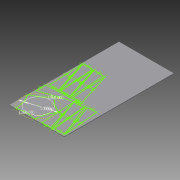
# Autodesk Inventor part: Birdhouse Board
Saved by Autodesk Inventor 2015 (Build 190159000, 159)
## iProperties
Created: 2018-03-09
Part Number: Birdhouse Board
Material: Generic
Document SubType Name: Modeling
Designer: Administrator
Density: 1 g/cm^3
Appearance: Default
Author: Administrator
Autodesk Inventor part; units mm, degrees
ref_plane "YZ Plane" through (0, 0, 0) normal (1, 0, 0) x (0, 1, 0)
ref_plane "XZ Plane" through (0, 0, 0) normal (0, 1, 0) x (-1, 0, 0)
ref_plane "XY Plane" through (0, 0, 0) normal (0, 0, 1) x (1, 0, 0)
sketch "Sketch1" plane through (0, 0, 0) normal (0, 1, 0) x (-1, 0, 0)
  line L0 (101.6, 169.3333) -> (-203.2, 169.3333)
  line L1 (-203.2, 169.3333) -> (-203.2, -440.2667)
  line L2 (-203.2, -440.2667) -> (101.6, -440.2667)
  line L3 (101.6, -440.2667) -> (101.6, 169.3333)
  point P0 (0, 0)
  dimension "d0" = 304.8
  dimension "d1" = 609.6
  constraints: 8 end point, 2 parallel, 1 horizontal, 1 perpendicular
  measures "d0" distance of L0.start L0.end
  measures "d1" distance of L0.end L1.end
extrude "Extrusion1" add sketch "Sketch1" along normal blind 3.175
sketch "Sketch2" plane through (0, 3.175, 0) normal (0, 1, 0) x (1, 0, 0)
  circle A0 centre (-15.875, -95.25) radius 63.5 construction
  circle A1 centre (-15.875, -95.25) radius 88.9 construction
  line L0 (-15.875, -6.35) -> (-53.1994, -43.8774)
  line L1 (-53.1994, -43.8774) -> (-100.4239, -67.7784)
  line L2 (-100.4239, -67.7784) -> (-76.2671, -114.8726)
  line L3 (-76.2671, -114.8726) -> (-68.1291, -167.1716)
  line L4 (-68.1291, -167.1716) -> (-15.875, -158.75)
  line L5 (36.3791, -167.1716) -> (-15.875, -158.75)
  line L6 (44.5171, -114.8726) -> (36.3791, -167.1716)
  line L7 (44.5171, -114.8726) -> (68.6739, -67.7784)
  line L8 (68.6739, -67.7784) -> (21.4494, -43.8774)
  line L9 (21.4494, -43.8774) -> (-15.875, -6.35)
  line L10 (122.7836, -165.1) -> (103.3018, -165.1)
  line L11 (103.3018, -168.275) -> (103.3018, -165.1)
  line L12 (95.6818, -168.275) -> (103.3018, -168.275)
  line L13 (95.6818, -165.1) -> (95.6818, -168.275)
  line L14 (73.025, -165.1) -> (95.6818, -165.1)
  line L15 (73.025, -165.1) -> (68.1796, -72.334)
  line L16 (68.1796, -72.334) -> (73.025, -165.1)
  line L17 (68.1796, -72.334) -> (71.3503, -72.1684)
  line L18 (71.3503, -72.1684) -> (70.9528, -64.5588)
  line L19 (70.9528, -64.5588) -> (71.3503, -72.1684)
  line L20 (70.9528, -64.5588) -> (67.7821, -64.7244)
  line L21 (67.7821, -64.7244) -> (70.9528, -64.5588)
  line L22 (67.7821, -64.7244) -> (63.2239, 22.5422)
  line L23 (67.7821, -64.7244) -> (63.2239, 22.5422)
  line L24 (63.2239, 22.5422) -> (90.9783, -64.8977)
  line L25 (90.9783, -64.8977) -> (63.2239, 22.5422)
  line L26 (90.9783, -64.8977) -> (87.9521, -65.8583)
  line L27 (87.9521, -65.8583) -> (90.2574, -73.1212)
  line L28 (90.2574, -73.1212) -> (93.2836, -72.1607)
  line L29 (90.2574, -73.1212) -> (93.2836, -72.1607)
  line L30 (93.2836, -72.1607) -> (122.7836, -165.1)
  line L31 (63.2239, 22.5422) -> (85.8673, 23.3211)
  line L32 (85.8673, 23.3211) -> (85.7582, 26.4942)
  line L33 (85.7582, 26.4942) -> (93.3737, 26.7562)
  line L34 (93.3737, 26.7562) -> (93.4828, 23.583)
  line L35 (93.4828, 23.583) -> (116.1262, 24.3619)
  line L36 (93.4828, 23.583) -> (116.1262, 24.3619)
  line L37 (116.1262, 24.3619) -> (124.1586, -68.1926)
  line L38 (124.1586, -68.1926) -> (116.1262, 24.3619)
  line L39 (124.1586, -68.1926) -> (127.3217, -67.9181)
  line L40 (127.3217, -67.9181) -> (127.9805, -75.5095)
  line L41 (127.3217, -67.9181) -> (127.9805, -75.5095)
  line L42 (127.9805, -75.5095) -> (124.8174, -75.784)
  line L43 (124.8174, -75.784) -> (132.8498, -168.3385)
  line L44 (124.8174, -75.784) -> (132.8498, -168.3385)
  line L45 (132.8498, -168.3385) -> (99.3425, -76.4774)
  line L46 (96.3597, -77.5654) -> (93.7485, -70.4068)
  line L47 (99.3425, -76.4774) -> (96.3597, -77.5654)
  line L48 (96.3597, -77.5654) -> (93.7485, -70.4068)
  line L49 (93.7485, -70.4068) -> (96.7313, -69.3188)
  line L50 (96.7313, -69.3188) -> (63.2239, 22.5422)
  line L51 (190.9567, -155.6753) -> (168.3382, -156.9913)
  line L52 (168.3382, -156.9913) -> (168.5226, -160.161)
  line L53 (168.5226, -160.161) -> (160.9155, -160.6036)
  line L54 (168.5226, -160.161) -> (160.9155, -160.6036)
  line L55 (160.9155, -160.6036) -> (160.731, -157.4339)
  line L56 (160.731, -157.4339) -> (138.1125, -158.75)
  line L57 (160.731, -157.4339) -> (138.1125, -158.75)
  line L58 (138.1125, -158.75) -> (127.8857, -66.4122)
  line L59 (127.8857, -66.4122) -> (138.1125, -158.75)
  line L60 (127.8857, -66.4122) -> (124.73, -66.7618)
  line L61 (124.73, -66.7618) -> (123.8912, -59.1881)
  line L62 (124.73, -66.7618) -> (123.8912, -59.1881)
  line L63 (123.8912, -59.1881) -> (127.0469, -58.8386)
  line L64 (127.0469, -58.8386) -> (116.8201, 33.4992)
  line L65 (127.0469, -58.8386) -> (116.8201, 33.4992)
  line L66 (116.8201, 33.4992) -> (152.4982, -57.5407)
  line L67 (155.4543, -56.3822) -> (158.2347, -63.4769)
  line L68 (152.4982, -57.5407) -> (155.4543, -56.3822)
  line L69 (155.4543, -56.3822) -> (158.2347, -63.4769)
  line L70 (158.2347, -63.4769) -> (155.2786, -64.6354)
  line L71 (155.2786, -64.6354) -> (190.9567, -155.6753)
  line L72 (155.2786, -64.6354) -> (190.9567, -155.6753)
  line L73 (190.9567, -155.6753) -> (168.3382, -156.9913)
  line L74 (168.3382, -156.9913) -> (168.5226, -160.161)
  line L75 (168.5226, -160.161) -> (160.9155, -160.6036)
  line L76 (168.5226, -160.161) -> (160.9155, -160.6036)
  line L77 (160.9155, -160.6036) -> (160.731, -157.4339)
  line L78 (160.731, -157.4339) -> (138.1125, -158.75)
  line L79 (160.731, -157.4339) -> (138.1125, -158.75)
  line L80 (138.1125, -158.75) -> (127.8857, -66.4122)
  line L81 (127.8857, -66.4122) -> (138.1125, -158.75)
  line L82 (127.8857, -66.4122) -> (124.73, -66.7618)
  line L83 (124.73, -66.7618) -> (123.8912, -59.1881)
  line L84 (124.73, -66.7618) -> (123.8912, -59.1881)
  line L85 (123.8912, -59.1881) -> (127.0469, -58.8386)
  line L86 (127.0469, -58.8386) -> (116.8201, 33.4992)
  line L87 (127.0469, -58.8386) -> (116.8201, 33.4992)
  line L88 (116.8201, 33.4992) -> (152.4982, -57.5407)
  line L89 (155.4543, -56.3822) -> (158.2347, -63.4769)
  line L90 (152.4982, -57.5407) -> (155.4543, -56.3822)
  line L91 (155.4543, -56.3822) -> (158.2347, -63.4769)
  line L92 (158.2347, -63.4769) -> (155.2786, -64.6354)
  line L93 (155.2786, -64.6354) -> (190.9567, -155.6753)
  line L94 (155.2786, -64.6354) -> (190.9567, -155.6753)
  line L95 (127, 34.925) -> (146.4644, 35.7476)
  line L96 (146.3304, 38.9198) -> (146.4644, 35.7476)
  line L97 (153.9436, 39.2415) -> (146.3304, 38.9198)
  line L98 (154.0776, 36.0694) -> (153.9436, 39.2415)
  line L99 (176.7142, 37.026) -> (154.0776, 36.0694)
  line L100 (176.7142, 37.026) -> (185.4723, -55.4526)
  line L101 (185.4723, -55.4526) -> (182.3115, -55.752)
  line L102 (182.3115, -55.752) -> (183.0299, -63.338)
  line L103 (183.0299, -63.338) -> (186.1907, -63.0387)
  line L104 (186.1907, -63.0387) -> (194.4296, -150.035)
  line L105 (194.4296, -150.035) -> (163.0079, -63.8449)
  line L106 (163.0079, -63.8449) -> (165.9908, -62.7575)
  line L107 (165.9908, -62.7575) -> (163.3809, -55.5984)
  line L108 (163.3809, -55.5984) -> (160.398, -56.6858)
  line L109 (160.398, -56.6858) -> (127, 34.925)
  line L110 (-37.5539, 39.6875) -> (-57.0357, 39.6875)
  line L111 (-57.0357, 36.5125) -> (-57.0357, 39.6875)
  line L112 (-64.6557, 36.5125) -> (-57.0357, 36.5125)
  line L113 (-64.6557, 39.6875) -> (-64.6557, 36.5125)
  line L114 (-87.3125, 39.6875) -> (-64.6557, 39.6875)
  line L115 (-87.3125, 39.6875) -> (-92.1579, 132.4535)
  line L116 (-92.1579, 132.4535) -> (-88.9872, 132.6191)
  line L117 (-88.9872, 132.6191) -> (-89.3847, 140.2287)
  line L118 (-89.3847, 140.2287) -> (-92.5554, 140.0631)
  line L119 (-92.5554, 140.0631) -> (-97.1136, 227.3297)
  line L120 (-97.1136, 227.3297) -> (-69.3592, 139.8898)
  line L121 (-69.3592, 139.8898) -> (-72.3854, 138.9292)
  line L122 (-72.3854, 138.9292) -> (-70.0801, 131.6663)
  line L123 (-70.0801, 131.6663) -> (-67.0539, 132.6268)
  line L124 (-67.0539, 132.6268) -> (-37.5539, 39.6875)
  line L125 (22.7711, 42.8625) -> (3.2893, 42.8625)
  line L126 (3.2893, 39.6875) -> (3.2893, 42.8625)
  line L127 (-4.3307, 39.6875) -> (3.2893, 39.6875)
  line L128 (-4.3307, 42.8625) -> (-4.3307, 39.6875)
  line L129 (-26.9875, 42.8625) -> (-4.3307, 42.8625)
  line L130 (-26.9875, 42.8625) -> (-31.8329, 135.6285)
  line L131 (-31.8329, 135.6285) -> (-28.6622, 135.7941)
  line L132 (-28.6622, 135.7941) -> (-29.0597, 143.4037)
  line L133 (-29.0597, 143.4037) -> (-32.2304, 143.2381)
  line L134 (-32.2304, 143.2381) -> (-36.7886, 230.5047)
  line L135 (-36.7886, 230.5047) -> (-9.0342, 143.0648)
  line L136 (-9.0342, 143.0648) -> (-12.0604, 142.1042)
  line L137 (-12.0604, 142.1042) -> (-9.7551, 134.8413)
  line L138 (-9.7551, 134.8413) -> (-6.7289, 135.8018)
  line L139 (-6.7289, 135.8018) -> (22.7711, 42.8625)
  line L140 (87.8586, 44.45) -> (68.3768, 44.45)
  line L141 (68.3768, 41.275) -> (68.3768, 44.45)
  line L142 (60.7568, 41.275) -> (68.3768, 41.275)
  line L143 (60.7568, 44.45) -> (60.7568, 41.275)
  line L144 (38.1, 44.45) -> (60.7568, 44.45)
  line L145 (38.1, 44.45) -> (33.2546, 137.216)
  line L146 (33.2546, 137.216) -> (36.4253, 137.3816)
  line L147 (36.4253, 137.3816) -> (36.0278, 144.9912)
  line L148 (36.0278, 144.9912) -> (32.8571, 144.8256)
  line L149 (32.8571, 144.8256) -> (28.2989, 232.0922)
  line L150 (28.2989, 232.0922) -> (56.0533, 144.6523)
  line L151 (56.0533, 144.6523) -> (53.0271, 143.6917)
  line L152 (53.0271, 143.6917) -> (55.3324, 136.4288)
  line L153 (55.3324, 136.4288) -> (58.3586, 137.3893)
  line L154 (58.3586, 137.3893) -> (87.8586, 44.45)
  line L155 (-96.8375, -25.4) -> (-96.8375, -2.7432)
  line L156 (-96.8375, -2.7432) -> (-100.0125, -2.7432)
  line L157 (-100.0125, -2.7432) -> (-100.0125, 4.8768)
  line L158 (-100.0125, -2.7432) -> (-100.0125, 4.8768)
  line L159 (-100.0125, 4.8768) -> (-96.8375, 4.8768)
  line L160 (-96.8375, 4.8768) -> (-96.8375, 27.5336)
  line L161 (-96.8375, 4.8768) -> (-96.8375, 27.5336)
  line L162 (-96.8375, 27.5336) -> (-4.0616, 32.3795)
  line L163 (-4.0616, 32.3795) -> (-96.8375, 27.5336)
  line L164 (-4.0616, 32.3795) -> (-4.2272, 35.5502)
  line L165 (-4.2272, 35.5502) -> (3.3824, 35.9477)
  line L166 (-4.2272, 35.5502) -> (3.3824, 35.9477)
  line L167 (3.3824, 35.9477) -> (3.548, 32.777)
  line L168 (3.548, 32.777) -> (96.3239, 37.623)
  line L169 (3.548, 32.777) -> (96.3239, 37.623)
  line L170 (96.3239, 37.623) -> (3.3653, 7.2933)
  line L171 (4.3501, 4.2749) -> (-2.8941, 1.9113)
  line L172 (3.3653, 7.2933) -> (4.3501, 4.2749)
  line L173 (4.3501, 4.2749) -> (-2.8941, 1.9113)
  line L174 (-2.8941, 1.9113) -> (-3.8789, 4.9297)
  line L175 (-3.8789, 4.9297) -> (-96.8375, -25.4)
  line L176 (-3.8789, 4.9297) -> (-96.8375, -25.4)
  line L177 (-96.8375, -25.4) -> (-96.8375, -2.7432)
  line L178 (-96.8375, -2.7432) -> (-100.0125, -2.7432)
  line L179 (-100.0125, -2.7432) -> (-100.0125, 4.8768)
  line L180 (-100.0125, -2.7432) -> (-100.0125, 4.8768)
  line L181 (-100.0125, 4.8768) -> (-96.8375, 4.8768)
  line L182 (-96.8375, 4.8768) -> (-96.8375, 27.5336)
  line L183 (-96.8375, 4.8768) -> (-96.8375, 27.5336)
  line L184 (-96.8375, 27.5336) -> (-4.0616, 32.3795)
  line L185 (-4.0616, 32.3795) -> (-96.8375, 27.5336)
  line L186 (-4.0616, 32.3795) -> (-4.2272, 35.5502)
  line L187 (-4.2272, 35.5502) -> (3.3824, 35.9477)
  line L188 (-4.2272, 35.5502) -> (3.3824, 35.9477)
  line L189 (3.3824, 35.9477) -> (3.548, 32.777)
  line L190 (3.548, 32.777) -> (96.3239, 37.623)
  line L191 (3.548, 32.777) -> (96.3239, 37.623)
  line L192 (96.3239, 37.623) -> (3.3653, 7.2933)
  line L193 (4.3501, 4.2749) -> (-2.8941, 1.9113)
  line L194 (3.3653, 7.2933) -> (4.3501, 4.2749)
  line L195 (4.3501, 4.2749) -> (-2.8941, 1.9113)
  line L196 (-2.8941, 1.9113) -> (-3.8789, 4.9297)
  line L197 (-3.8789, 4.9297) -> (-96.8375, -25.4)
  line L198 (-3.8789, 4.9297) -> (-96.8375, -25.4)
  line L199 (-95.25, 233.3625) -> (-72.5932, 233.3625)
  line L200 (-72.5932, 233.3625) -> (-72.5932, 236.5375)
  line L201 (-72.5932, 236.5375) -> (-64.9732, 236.5375)
  line L202 (-72.5932, 236.5375) -> (-64.9732, 236.5375)
  line L203 (-64.9732, 236.5375) -> (-64.9732, 233.3625)
  line L204 (-64.9732, 233.3625) -> (-42.3164, 233.3625)
  line L205 (-64.9732, 233.3625) -> (-42.3164, 233.3625)
  line L206 (-42.3164, 233.3625) -> (-37.4705, 140.5866)
  line L207 (-37.4705, 140.5866) -> (-42.3164, 233.3625)
  line L208 (-37.4705, 140.5866) -> (-34.2998, 140.7522)
  line L209 (-34.2998, 140.7522) -> (-33.9023, 133.1426)
  line L210 (-34.2998, 140.7522) -> (-33.9023, 133.1426)
  line L211 (-33.9023, 133.1426) -> (-37.073, 132.977)
  line L212 (-37.073, 132.977) -> (-32.227, 40.2011)
  line L213 (-37.073, 132.977) -> (-32.227, 40.2011)
  line L214 (-32.227, 40.2011) -> (-62.5567, 133.1597)
  line L215 (-65.5751, 132.1749) -> (-67.9387, 139.4191)
  line L216 (-62.5567, 133.1597) -> (-65.5751, 132.1749)
  line L217 (-65.5751, 132.1749) -> (-67.9387, 139.4191)
  line L218 (-67.9387, 139.4191) -> (-64.9203, 140.4039)
  line L219 (-64.9203, 140.4039) -> (-95.25, 233.3625)
  line L220 (-64.9203, 140.4039) -> (-95.25, 233.3625)
  line L221 (-95.25, 233.3625) -> (-72.5932, 233.3625)
  line L222 (-72.5932, 233.3625) -> (-72.5932, 236.5375)
  line L223 (-72.5932, 236.5375) -> (-64.9732, 236.5375)
  line L224 (-72.5932, 236.5375) -> (-64.9732, 236.5375)
  line L225 (-64.9732, 236.5375) -> (-64.9732, 233.3625)
  line L226 (-64.9732, 233.3625) -> (-42.3164, 233.3625)
  line L227 (-64.9732, 233.3625) -> (-42.3164, 233.3625)
  line L228 (-42.3164, 233.3625) -> (-37.4705, 140.5866)
  line L229 (-37.4705, 140.5866) -> (-42.3164, 233.3625)
  line L230 (-37.4705, 140.5866) -> (-34.2998, 140.7522)
  line L231 (-34.2998, 140.7522) -> (-33.9023, 133.1426)
  line L232 (-34.2998, 140.7522) -> (-33.9023, 133.1426)
  line L233 (-33.9023, 133.1426) -> (-37.073, 132.977)
  line L234 (-37.073, 132.977) -> (-32.227, 40.2011)
  line L235 (-37.073, 132.977) -> (-32.227, 40.2011)
  line L236 (-32.227, 40.2011) -> (-62.5567, 133.1597)
  line L237 (-65.5751, 132.1749) -> (-67.9387, 139.4191)
  line L238 (-62.5567, 133.1597) -> (-65.5751, 132.1749)
  line L239 (-65.5751, 132.1749) -> (-67.9387, 139.4191)
  line L240 (-67.9387, 139.4191) -> (-64.9203, 140.4039)
  line L241 (-64.9203, 140.4039) -> (-95.25, 233.3625)
  line L242 (-64.9203, 140.4039) -> (-95.25, 233.3625)
  line L243 (-32.8605, 231.2614) -> (-10.2037, 231.2614)
  line L244 (-10.2037, 231.2614) -> (-10.2037, 234.4364)
  line L245 (-10.2037, 234.4364) -> (-2.5837, 234.4364)
  line L246 (-10.2037, 234.4364) -> (-2.5837, 234.4364)
  line L247 (-2.5837, 234.4364) -> (-2.5837, 231.2614)
  line L248 (-2.5837, 231.2614) -> (20.0731, 231.2614)
  line L249 (-2.5837, 231.2614) -> (20.0731, 231.2614)
  line L250 (20.0731, 231.2614) -> (24.9191, 138.4855)
  line L251 (24.9191, 138.4855) -> (20.0731, 231.2614)
  line L252 (24.9191, 138.4855) -> (28.0898, 138.6511)
  line L253 (28.0898, 138.6511) -> (28.4872, 131.0415)
  line L254 (28.0898, 138.6511) -> (28.4872, 131.0415)
  line L255 (28.4872, 131.0415) -> (25.3166, 130.8759)
  line L256 (25.3166, 130.8759) -> (30.1625, 38.1)
  line L257 (30.1625, 38.1) -> (-0.1672, 131.0586)
  line L258 (-3.1856, 130.0738) -> (-5.5492, 137.318)
  line L259 (-0.1672, 131.0586) -> (-3.1856, 130.0738)
  line L260 (-3.1856, 130.0738) -> (-5.5492, 137.318)
  line L261 (-5.5492, 137.318) -> (-2.5308, 138.3028)
  line L262 (-2.5308, 138.3028) -> (-32.8605, 231.2614)
  line L263 (-2.5308, 138.3028) -> (-32.8605, 231.2614)
  line L264 (-32.8605, 231.2614) -> (-10.2037, 231.2614)
  line L265 (-10.2037, 231.2614) -> (-10.2037, 234.4364)
  line L266 (-10.2037, 234.4364) -> (-2.5837, 234.4364)
  line L267 (-10.2037, 234.4364) -> (-2.5837, 234.4364)
  line L268 (-2.5837, 234.4364) -> (-2.5837, 231.2614)
  line L269 (-2.5837, 231.2614) -> (20.0731, 231.2614)
  line L270 (-2.5837, 231.2614) -> (20.0731, 231.2614)
  line L271 (20.0731, 231.2614) -> (24.9191, 138.4855)
  line L272 (24.9191, 138.4855) -> (20.0731, 231.2614)
  line L273 (24.9191, 138.4855) -> (28.0898, 138.6511)
  line L274 (28.0898, 138.6511) -> (28.4872, 131.0415)
  line L275 (28.0898, 138.6511) -> (28.4872, 131.0415)
  line L276 (28.4872, 131.0415) -> (25.3166, 130.8759)
  line L277 (-3.1856, 130.0738) -> (-5.5492, 137.318)
  line L278 (-0.1672, 131.0586) -> (-3.1856, 130.0738)
  line L279 (-3.1856, 130.0738) -> (-5.5492, 137.318)
  line L280 (-5.5492, 137.318) -> (-2.5308, 138.3028)
  line L281 (-2.5308, 138.3028) -> (-32.8605, 231.2614)
  line L282 (-2.5308, 138.3028) -> (-32.8605, 231.2614)
  point P0 (0, 0)
  dimension "d8" = 127
  dimension "d9" = 177.8
  dimension "d10" = 360
  dimension "d11" = 360
  constraints: 566 end point, 82 perpendicular, 56 collinear, 8 parallel, 2 coincident, 2 vertical, 2 vertical alignment, 16 other
sketch "Sketch3" plane through (0, 3.175, 0) normal (0, 1, 0) x (1, 0, 0)
  point P0 (0, 0)
body "Solid1"
